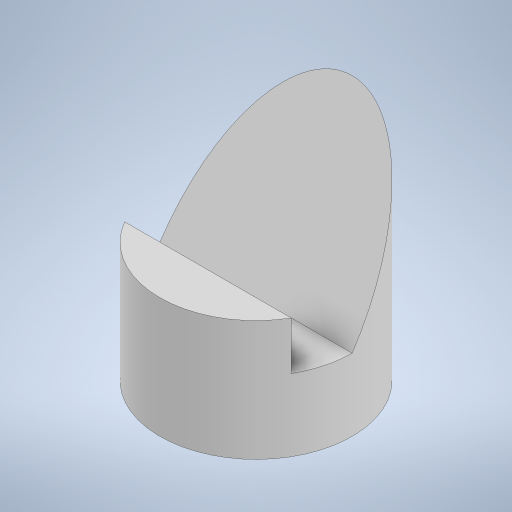
# Autodesk Inventor part: Цилиндр с вырезом
Saved by Autodesk Inventor 2023.2 (Build 272271030, 271C)
## iProperties
Created: 2023-09-29
Part Number: Цилиндр с вырезом
Material: Типовые
Document SubType Name: Modeling
Designer: User
Density: 1 g/cm^3
Appearance: По умолчанию
Author: User
Autodesk Inventor part; units mm, degrees
ref_plane "YZ Plane" through (0, 0, 0) normal (1, 0, 0) x (0, 1, 0)
ref_plane "XZ Plane" through (0, 0, 0) normal (0, 1, 0) x (-1, 0, 0)
ref_plane "XY Plane" through (0, 0, 0) normal (0, 0, 1) x (1, 0, 0)
sketch "Эскиз1" plane through (0, 0, 0) normal (0, 1, 0) x (-1, 0, 0)
  circle A0 centre (0, 0) radius 40
  dimension "d0" = 80
  constraints: 1 centre point, 1 coincident
  measures "d0" diameter of A0
extrude "Выдавливание1" add sketch "Эскиз1" along normal blind 90
sketch "Эскиз2" plane through (0, 0, 0) normal (1, 0, 0) x (0, 1, 0)
  line L0 (90, -40) -> (90, 40) projected
  line L1 (90, -40) -> (30, 0)
  line L2 (30, 0) -> (30, 20)
  line L3 (30, 20) -> (50, 20)
  line L4 (50, 20) -> (50, 40.1134)
  point P0 (0, 0)
  dimension "d3" = 60
  dimension "d4" = 20
  dimension "d5" = 20
  constraints: 8 end point, 2 perpendicular, 1 vertical
  measures "d3" horizontal distance of L1.end L0.start
  measures "d4" distance of L1.end L2.end
  measures "d5" distance of L2.end L3.end
extrude "Выдавливание2" cut sketch "Эскиз2" along normal mid plane 90 fills toward (50.05, 30.0567) open curves L4 L3 L2 L1 L0
